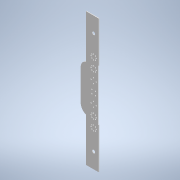
# Autodesk Inventor part: plate1
Saved by Autodesk Inventor 2020.1 (Build 241239000, 239)
## iProperties
Created: 2019-12-06
Part Number: plate1
Material: Generic
Document SubType Name: Modeling
Designer: tbloo
Density: 1 g/cm^3
Appearance: Default
Author: tbloo
Autodesk Inventor part; units mm, degrees
ref_plane "YZ Plane" through (0, 0, 0) normal (1, 0, 0) x (0, 1, 0)
ref_plane "XZ Plane" through (0, 0, 0) normal (0, 1, 0) x (-1, 0, 0)
ref_plane "XY Plane" through (0, 0, 0) normal (0, 0, 1) x (1, 0, 0)
sketch "Sketch1" plane through (0, 0, 0) normal (0, 0, 1) x (1, 0, 0)
  circle A0 centre (32, -32) radius 4.7
  circle A1 centre (32, -352) radius 4.7
  line L0 (48, -272) -> (48, -398)
  arc A2 (46, -400) -> (48, -398) centre (46, -398) ccw
  line L1 (46, -400) -> (8, -400)
  line L2 (48, 14) -> (48, -112)
  line L3 (8, 16) -> (46, 16)
  arc A3 (48, 14) -> (46, 16) centre (46, 14) ccw
  circle A4 centre (32, -120) radius 1.85
  circle A5 centre (37.6569, -122.3431) radius 1.85
  circle A6 centre (40, -128) radius 1.85
  circle A7 centre (37.6569, -133.6569) radius 1.85
  circle A8 centre (32, -136) radius 1.85
  circle A9 centre (26.3431, -133.6569) radius 1.85
  circle A10 centre (23.8856, -128.1676) radius 1.85
  circle A11 centre (26.3431, -122.3431) radius 1.85
  circle A12 centre (32, -152) radius 1.85
  circle A13 centre (40, -160) radius 1.85
  circle A14 centre (24, -160) radius 1.85
  circle A15 centre (32, -168) radius 1.85
  circle A16 centre (37.6569, -186.3431) radius 1.85
  circle A17 centre (37.6569, -197.6569) radius 1.85
  circle A18 centre (26.3431, -186.3431) radius 1.85
  circle A19 centre (26.3431, -197.6569) radius 1.85
  circle A20 centre (32, -216) radius 1.85
  circle A21 centre (40, -224) radius 1.85
  circle A22 centre (32, -232) radius 1.85
  circle A23 centre (24, -224) radius 1.85
  circle A24 centre (32, -248) radius 1.85
  circle A25 centre (37.6569, -250.3431) radius 1.85
  circle A26 centre (40, -256) radius 1.85
  circle A27 centre (37.6569, -261.6569) radius 1.85
  circle A28 centre (32, -264) radius 1.85
  circle A29 centre (26.3431, -261.6569) radius 1.85
  circle A30 centre (24, -256) radius 1.85
  circle A31 centre (26.3431, -250.3431) radius 1.85
  circle A32 centre (37.6569, -101.6569) radius 1.85
  circle A33 centre (40, -96) radius 1.85
  circle A34 centre (37.6569, -90.3431) radius 1.85
  circle A35 centre (32, -88) radius 1.85
  circle A36 centre (26.3431, -90.3431) radius 1.85
  circle A37 centre (24, -96) radius 1.85
  circle A38 centre (26.3431, -101.6569) radius 1.85
  circle A39 centre (32, -104) radius 1.85
  circle A40 centre (24, -288.0038) radius 1.85
  circle A41 centre (26.3431, -293.6606) radius 1.85
  circle A42 centre (32, -296.0038) radius 1.85
  circle A43 centre (37.6569, -293.6606) radius 1.85
  circle A44 centre (40, -288.0038) radius 1.85
  circle A45 centre (37.6569, -282.3469) radius 1.85
  circle A46 centre (32, -280.0038) radius 1.85
  circle A47 centre (26.3431, -282.3469) radius 1.85
  line L4 (48, -272) -> (46, -272)
  line L5 (46, -112) -> (48, -112)
  line L6 (46, -112) -> (46, -272)
  line L7 (8, -120.2479) -> (8, 16)
  arc A48 (8, -120.2479) -> (-8.4, -144) centre (17, -144) ccw
  line L8 (-8.4, -240) -> (-8.4, -144)
  arc A49 (-8.4, -240) -> (8, -263.7521) centre (17, -240) ccw
  line L9 (8, -400) -> (8, -263.7521)
  point P0 (0, 0)
  point P1 (48, -114.5)
  constraints: 50 centre point, 20 end point, 8 point on circle, 3 vertical, 10 other
extrude "Extrusion1" add sketch "Sketch1" along normal blind 2
body "Solid1"
